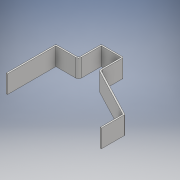
# Autodesk Inventor part: INTERNAL FRAME
Saved by Autodesk Inventor 2018 (Build 220112000, 112)
## iProperties
Created: 2018-10-15
Part Number: INTERNAL FRAME
Material: Genérico
Document SubType Name: Modeling
Designer: Toshiba
Density: 1 g/cm^3
Appearance: Valor por defecto
Author: Toshiba
Autodesk Inventor part; units mm, degrees
ref_plane "YZ Plane" through (0, 0, 0) normal (1, 0, 0) x (0, 1, 0)
ref_plane "XZ Plane" through (0, 0, 0) normal (0, 1, 0) x (-1, 0, 0)
ref_plane "XY Plane" through (0, 0, 0) normal (0, 0, 1) x (1, 0, 0)
sketch "Boceto1" plane through (0, 0, 0) normal (0, 0, 1) x (1, 0, 0)
  line L0 (200, -104) -> (200, -8.6304)
  arc A0 (200, -8.6304) -> (196.784, -3.3155) centre (194, -8.6304) ccw
  line L1 (196.784, -3.3155) -> (-6.784, 103.3155)
  arc A1 (-10, 108.6304) -> (-6.784, 103.3155) centre (-4, 108.6304) ccw
  line L2 (-10, 108.6304) -> (-10, 194)
  arc A2 (-10, 194) -> (-16, 200) centre (-16, 194) ccw
  line L3 (-16, 200) -> (-99, 200)
  arc A3 (-99, 200) -> (-105, 194) centre (-99, 194) ccw
  line L4 (-105, 194) -> (-105, 111)
  arc A4 (-111, 105) -> (-105, 111) centre (-111, 111) ccw
  line L5 (-111, 105) -> (-194, 105)
  arc A5 (-194, 105) -> (-200, 99) centre (-194, 99) ccw
  line L6 (-200, 99) -> (-200, -104)
  line L7 (-194, -104) -> (-194, 99)
  line L8 (-194, 99) -> (-111, 99)
  arc A6 (-111, 99) -> (-99, 111) centre (-111, 111) ccw
  line L9 (-99, 111) -> (-99, 194)
  line L10 (-99, 194) -> (-16, 194)
  line L11 (-16, 194) -> (-16, 108.6304)
  arc A7 (-16, 108.6304) -> (-9.5681, 98.0005) centre (-4, 108.6304) ccw
  line L12 (-9.5681, 98.0005) -> (194, -8.6304)
  line L13 (194, -8.6304) -> (194, -104)
  line L14 (-200, -104) -> (-194, -104)
  line L15 (194, -104) -> (200, -104)
  point P0 (0, 0)
  point P1 (0, 0)
  dimension "d0" = 6
  constraints: 32 end point, 16 point on circle, 8 centre point, 1 collinear, 1 horizontal, 8 other
  measures "d0" distance between parallel lines of L4 L9
extrude "Extrusión1" add sketch "Boceto1" along normal mid plane 75
